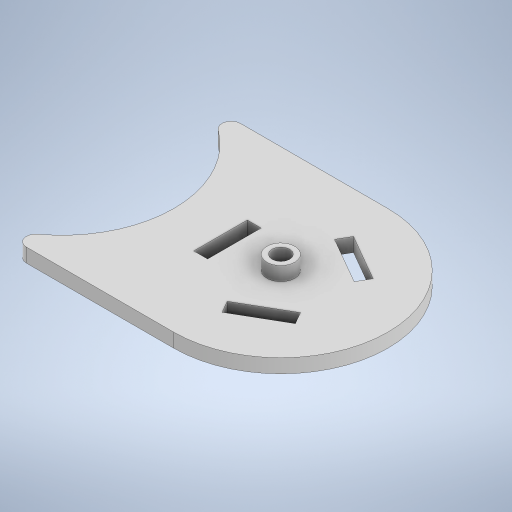
# Autodesk Inventor part: ベルト_bush_upper
Saved by Autodesk Inventor 2024.1 (Build 281209000, 209)
## iProperties
Created: 2024-03-27
Part Number: ベルト_bush_upper
Material: 一般
Document SubType Name: Modeling
Designer: hibik
Density: 1 g/cm^3
Appearance: 既定
Author: hibik
Autodesk Inventor part; units mm, degrees
ref_plane "YZ Plane" through (0, 0, 0) normal (1, 0, 0) x (0, 1, 0)
ref_plane "XZ Plane" through (0, 0, 0) normal (0, 1, 0) x (-1, 0, 0)
ref_plane "XY Plane" through (0, 0, 0) normal (0, 0, 1) x (1, 0, 0)
sketch "スケッチ1" plane through (0, 0, 0) normal (0, 1, 0) x (-1, 0, 0)
  circle A0 centre (0, 0) radius 6
  dimension "d0" = 12
  constraints: 1 centre point, 1 coincident
  measures "d0" diameter of A0
extrude "押し出し1" add sketch "スケッチ1" along normal blind 1
sketch "スケッチ2" plane through (0, 1, 0) normal (0, 1, 0) x (1, 0, 0)
  circle A0 centre (0, 0) radius 3
  dimension "d3" = 6
  constraints: 1 centre point, 1 coincident
  measures "d3" diameter of A0
extrude "押し出し2" add sketch "スケッチ2" along normal blind 3
sketch "スケッチ3" plane through (0, 4, 0) normal (0, 1, 0) x (1, 0, 0)
  circle A0 centre (0, 0) radius 1.9
  dimension "d6" = 3.8
  constraints: 1 centre point, 1 coincident
  measures "d6" diameter of A0
extrude "押し出し3" cut sketch "スケッチ3" against normal through all
sketch "スケッチ4" plane through (0, 1, 0) normal (0, 1, 0) x (1, 0, 0)
  circle A0 centre (0, 0) radius 23.55
  circle A1 centre (-47.1, 0) radius 23.55
  line L0 (-47.1, 23.55) -> (0, 23.55)
  line L1 (0, -23.55) -> (-47.1, -23.55)
  circle A2 centre (0, 0) radius 1.9 projected
  dimension "d11" = 47.1
  constraints: 4 end point, 4 point on circle, 4 tangent, 2 centre point, 1 coincident, 1 equal radius, 1 horizontal alignment, 1 parallel
  measures "d11" distance of point (0, 0) A1.centre
extrude "押し出し4" add sketch "スケッチ4" against normal blind 3 contours A0 | A0 A1 L0 | L1 A1 A0
sketch "スケッチ5" plane through (0, -2, 0) normal (0, -1, 0) x (1, 0, 0)
  circle A0 centre (0, 0) radius 23.05
  circle A1 centre (-47.1, 0) radius 24.05
  arc A2 (0, -23.55) -> (0, 23.55) centre (0, 0) ccw projected
  arc A3 (-47.1, -23.55) -> (-47.1, 23.55) centre (-47.1, 0) ccw projected
  line L0 (0, 23.05) -> (-40.2371, 23.05)
  line L1 (0, -23.05) -> (-40.2371, -23.05)
  line L2 (30, 40) -> (-80, 40)
  line L3 (-80, 40) -> (-80, -50)
  line L4 (-80, -50) -> (30, -50)
  line L5 (30, -50) -> (30, 40)
  dimension "d14" = 0.5
  dimension "d15" = 0.5
  constraints: 12 end point, 4 point on circle, 3 horizontal, 2 centre point, 2 concentric, 2 parallel, 2 tangent, 1 coincident, 1 perpendicular
  measures "d14" radial gap between concentric circles of A2 A0
  measures "d15" radial gap between concentric circles of A3 A1
extrude "押し出し5" cut sketch "スケッチ5" against normal through all contours A1 | L5 L4 L3 L2
fillet "フィレット1" radius 2 2 edges at (-40.2371, -0.5, 23.05) (-40.2371, -0.5, -23.05)
sketch "スケッチ6" plane through (0, -2, 0) normal (0, -1, 0) x (1, 0, 0)
  circle A0 centre (0, 0) radius 10
  line L0 (10, 5.7735) -> (10, -5.7735)
  line L1 (10, -5.7735) -> (0, -11.547)
  line L2 (0, -11.547) -> (-10, -5.7735)
  line L3 (-10, -5.7735) -> (-10, 5.7735)
  line L4 (-10, 5.7735) -> (0, 11.547)
  line L5 (0, 11.547) -> (10, 5.7735)
  line L6 (-10, -5.7735) -> (-10, 5.7735)
  line L7 (-10, 5.7735) -> (-13, 5.7735)
  line L8 (-13, 5.7735) -> (-13, -5.7735)
  line L9 (-13, -5.7735) -> (-10, -5.7735)
  line L10 (0, 11.547) -> (10, 5.7735)
  line L11 (10, 5.7735) -> (11.5, 8.3716)
  line L12 (11.5, 8.3716) -> (1.5, 14.1451)
  line L13 (1.5, 14.1451) -> (0, 11.547)
  line L14 (10, -5.7735) -> (0, -11.547)
  line L15 (0, -11.547) -> (1.5, -14.1451)
  line L16 (1.5, -14.1451) -> (11.5, -8.3716)
  line L17 (11.5, -8.3716) -> (10, -5.7735)
  point P0 (10, -5.7735)
  dimension "d19" = 20
  dimension "d20" = 3
  dimension "d21" = 3
  dimension "d22" = 3
  constraints: 36 end point, 7 equal length, 3 perpendicular, 2 coincident, 1 centre point, 1 collinear, 1 point on line, 1 tangent, 1 vertical, 13 other
  measures "d19" diameter of A0
  measures "d20" distance of L7.end L3.end
  measures "d21" distance of L11.end L0.start
  measures "d22" distance of L15.end L1.end
extrude "押し出し6" cut sketch "スケッチ6" against normal through all contours L5 L13 L12 L11 | L1 L17 L16 L15 | L3 L9 L8 L7
